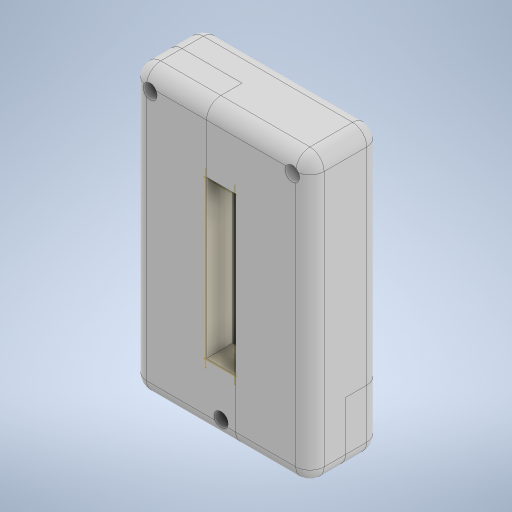
# Autodesk Inventor part: LYSO-holder-V3
Saved by Autodesk Inventor 2023 (Build 270158000, 158)
## iProperties
Created: 2023-09-07
Part Number: LYSO-holder-V3
Material: Generic
Document SubType Name: Modeling
Designer: AxLab
Density: 1 g/cm^3
Appearance: Default
Author: AxLab
## iProperties of the stored document LYSO-holder-V3_3DPrint.ipt
Created: 2023-12-19
Part Number: LYSO-holder-V3_3DPrint
Material: Generic
Document SubType Name: Modeling
Designer: AxLab
Density: 1 g/cm^3
Appearance: Default
Author: AxLab
Autodesk Inventor part; units mm, degrees
ref_plane "YZ Plane" through (0, 0, 0) normal (1, 0, 0) x (0, 1, 0)
ref_plane "XZ Plane" through (0, 0, 0) normal (0, 1, 0) x (-1, 0, 0)
ref_plane "XY Plane" through (0, 0, 0) normal (0, 0, 1) x (1, 0, 0)
sketch "Sketch1" plane through (0, 0, 0) normal (0, 0, 1) x (1, 0, 0)
  line L0 (-12.5, -20) -> (12.5, -20)
  line L1 (12.5, -20) -> (12.5, 20)
  line L2 (12.5, 20) -> (-12.5, 20)
  line L3 (-12.5, 20) -> (-12.5, -20)
  line L4 (-12.5, -20) -> (12.5, 20) construction
  line L5 (12.5, -20) -> (-12.5, 20) construction
  line L6 (-5, -20) -> (5, -20)
  line L7 (5, -20) -> (5, 20)
  line L8 (5, 20) -> (-5, 20)
  line L9 (-5, 20) -> (-5, -20)
  line L10 (-5, -20) -> (5, 20) construction
  line L11 (5, -20) -> (-5, 20) construction
  line L12 (-12.5, 20) -> (12.5, 20)
  line L13 (12.5, 20) -> (12.5, 10)
  line L14 (12.5, 10) -> (-12.5, 10)
  line L15 (-12.5, 10) -> (-12.5, 20)
  line L16 (-12.5, 20) -> (-10, 20)
  line L17 (-10, 20) -> (-10, 17.5)
  line L18 (-10, 17.5) -> (-12.5, 17.5)
  line L19 (-12.5, 17.5) -> (-12.5, 20)
  circle A0 centre (-10, 17.5) radius 1
  line L20 (0, 20) -> (0, -20)
  circle A1 centre (10, 17.5) radius 1
  line L21 (0, -20) -> (0, -17.5)
  circle A2 centre (0, -17.5) radius 1
  point P0 (0, 0)
  point P1 (5, 10)
  point P2 (-5, 10)
  dimension "d0" = 25
  dimension "d1" = 40
  dimension "d2" = 10
  dimension "d3" = 10
  dimension "d4" = 2.5
  dimension "d5" = 2.5
  dimension "d6" = 2
  dimension "d7" = 2.5
  dimension "d8" = 2
  constraints: 44 end point, 8 parallel, 6 midpoint, 4 horizontal, 4 perpendicular, 3 centre point, 3 point on line, 2 coincident, 1 symmetric about line, 1 other
  measures "d0" distance of L2.end L1.end
  measures "d1" distance of L1.end L0.end
  measures "d2" distance of L8.end L7.end
  measures "d3" distance of L12.end L13.end
  measures "d4" distance of L17.end L18.end
  measures "d5" distance of L16.end L17.end
  measures "d6" diameter of A0
  measures "d7" distance of L20.end L21.end
  measures "d8" diameter of A2
extrude "Extrusion1" add sketch "Sketch1" along normal blind 10 contours L3 L14 L9 L0 | L9 L14 L20 A2 L0 | L3 L18 A0 L17 L2 L9 L14 | L20 A2 L14 L7 L0 | L9 L2 L20 L14 | L3 L2 L17 A0 L18 | L7 L14 L1 L0 | A2 L20 | L20 A2 | L20 L2 L7 L14 | A0 L17 L18 | L18 L17 A0 | L7 L2 L1 L14 | A1
sketch "Sketch2" plane through (0, 0, 10) normal (0, 0, 1) x (1, 0, 0)
  line L0 (-2.05, -11.05) -> (2.05, -11.05)
  line L1 (2.05, -11.05) -> (2.05, 11.05)
  line L2 (2.05, 11.05) -> (-2.05, 11.05)
  line L3 (-2.05, 11.05) -> (-2.05, -11.05)
  line L4 (-2.05, -11.05) -> (2.05, 11.05) construction
  line L5 (2.05, -11.05) -> (-2.05, 11.05) construction
  point P0 (0, 0)
  dimension "d14" = 4.1
  dimension "d15" = 22.1
  constraints: 12 end point, 2 midpoint, 2 parallel, 1 horizontal, 1 perpendicular
  measures "d14" distance of L2.end L1.end
  measures "d15" distance of L1.end L0.end
extrude "Extrusion3" cut sketch "Sketch2" against normal blind 3.7
ref_plane "Work Plane1" through (-2.05, -11.05, 10) normal (1, 0, 0) x (0, 0, -1)
ref_plane "Work Plane2" through (-2.05, -11.05, 10) normal (0, 1, 0) x (1, 0, 0)
ref_plane "Work Plane6" through (-2.05, 11.05, 10) normal (0, -1, 0) x (1, 0, 0)
ref_plane "Work Plane7" through (0, 0, 5) normal (0, 0, 1) x (1, 0, 0)
ref_plane "Work Plane9" through (2.05, -11.05, 10) normal (-1, 0, 0) x (0, 0, 1)
split body "Split26" result two bodies by plane through (-2.05, -11.05, 10) normal (0, 1, 0) first body at (-4.1667, 9.65, 0.5)
split body "Split27" result two bodies by plane through (-2.05, -11.05, 10) normal (1, 0, 0) bodies 2 first body at (2.8, -0.7, 0.5)
split body "Split28" result two bodies by plane through (2.05, -11.05, 10) normal (-1, 0, 0) bodies 3 first body at (-7.65, -19.5, 6.6667)
split body "Split29" result two bodies by plane through (0, 0, 5) normal (0, 0, 1) bodies 5 first body at (-9.0167, 6.6667, 9.5)
split body "Split30" result two bodies by plane through (0, 0, 5) normal (0, 0, 1) bodies 7 first body at (5.5333, -14.0333, 5.5)
combine bodies "Combine14" operation type add bodies to combine 6 8 11
combine bodies "Combine15" operation type add bodies to combine 10 4 9
fillet "Fillet5" radius 2 18 edges at (-7.275, 20, 10) (-12.5, 20, 7.5) (-12.5, 0, 10) (-5.225, -20, 10) (12.5, -20, 2.5) (12.5, -15.525, 0) (0, -20, 0) (-12.5, -20, 5) (-12.5, -15.525, 0) (5.225, 20, 10) (12.5, 20, 5) (0, 20, 0) (-12.5, 20, 2.5) (7.275, -20, 10) (12.5, -20, 7.5) (12.5, 0, 10) (12.5, 4.475, 0) (-12.5, 4.475, 0)
sketch "Sketch13" plane through (-2.05, 11.05, 10) normal (0, 0, 1) x (1, 0, 0)
  line L0 (-8.45, -29.05) -> (-8.45, 6.95) projected
  line L1 (-8.45, 6.95) -> (-7.95, 6.95)
  line L2 (-7.95, 6.95) -> (-7.95, 6.45)
  line L3 (-7.95, 6.45) -> (-8.45, 6.45)
  line L4 (-8.45, 6.45) -> (-8.45, 6.95)
  line L5 (12.55, -22.1) -> (12.55, 6.95) projected
  line L6 (12.55, 6.95) -> (12.05, 6.95)
  line L7 (12.05, 6.95) -> (12.05, 6.45)
  line L8 (12.05, 6.45) -> (12.55, 6.45)
  line L9 (12.55, 6.45) -> (12.55, 6.95)
  line L10 (4.1, -22.1) -> (0, -22.1) projected
  line L11 (2.05, -22.1) -> (2.05, -29.05)
  line L12 (-8.45, -29.05) -> (12.55, -29.05) projected
  line L13 (2.05, -29.05) -> (2.05, -28.55)
  circle A0 centre (-7.95, 6.45) radius 1
  circle A1 centre (12.05, 6.45) radius 1
  circle A2 centre (2.05, -28.55) radius 1
  point P0 (2.05, -11.05)
  dimension "d88" = 0.5
  dimension "d89" = 0.5
  dimension "d90" = 0.5
  dimension "d91" = 0.5
  dimension "d92" = 0.5
  dimension "d93" = 2
  dimension "d94" = 2
  dimension "d95" = 2
  constraints: 20 end point, 4 parallel, 3 centre point, 3 coincident, 2 horizontal, 2 midpoint, 2 perpendicular, 1 point on line
  measures "d88" distance of L2.end L3.end
  measures "d89" distance of L1.end L2.end
  measures "d90" distance of L8.end L7.end
  measures "d91" distance of L7.end L6.end
  measures "d92" distance of L11.end L13.end
  measures "d93" diameter of A0
  measures "d94" diameter of A1
  measures "d95" diameter of A2
extrude "Extrusion11" cut sketch "Sketch13" against normal blind 11 contours L0 L1 L2 L3 | L8 L7 L6 L5 | L11 A2 L12 | L11 L12 A2 | L12 A2 | A0 | A1 bodies 10 6
body "Solid56"
body "Solid60"
